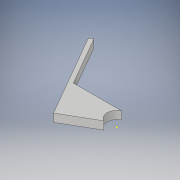
# Autodesk Inventor part: flipper-hug-left
Saved by Autodesk Inventor 2017 (Build 210142000, 142)
## iProperties
Created: 2017-02-21
Part Number: flipper-hug-left
Material: Generic
Document SubType Name: Modeling
Designer: John
Density: 1 g/cm^3
Appearance: Default
Author: John
Autodesk Inventor part; units mm, degrees
ref_plane "YZ Plane" through (0, 0, 0) normal (1, 0, 0) x (0, 1, 0)
ref_plane "XZ Plane" through (0, 0, 0) normal (0, 1, 0) x (-1, 0, 0)
ref_plane "XY Plane" through (0, 0, 0) normal (0, 0, 1) x (1, 0, 0)
sketch "Sketch1" plane through (0, 0, 0) normal (0, 1, 0) x (-1, 0, 0)
  point P0 (0, 0)
sketch "Sketch2" plane through (0, 0, 0) normal (0, 1, 0) x (-1, 0, 0)
  circle A0 centre (0, 0) radius 10 construction
  arc A1 (5.0714, -10.8757) -> (5.0714, 10.8757) centre (0, 0) ccw
  line L0 (5.0714, 10.8757) -> (5.0714, -10.8757) construction
  line L1 (5.0714, 10.8757) -> (26.8228, 10.8757) construction
  line L2 (5.0714, -10.8757) -> (65.0714, -10.8757)
  line L3 (5.0714, -10.8757) -> (65.0714, -10.8757) construction
  line L4 (65.0714, -10.8757) -> (100.0714, -71.4975)
  line L5 (100.0714, -71.4975) -> (104.4015, -68.9975)
  line L6 (5.0714, 10.8757) -> (58.2868, 10.8757)
  line L7 (58.2868, 10.8757) -> (104.4015, -68.9975)
  dimension "d0" = 20
  dimension "d1" = 90
  dimension "d2" = 2
  dimension "d3" = 130
  dimension "d4" = 60
  dimension "d5" = 0
  dimension "d6" = 70
  dimension "d7" = 120
  dimension "d8" = 5
  constraints: 16 end point, 3 horizontal, 2 centre point, 2 equal length, 2 point on circle, 1 coincident, 1 concentric, 1 parallel, 1 perpendicular, 1 point on line
  measures "d0" diameter of A0
  measures "d1" angle of L0 L1
  measures "d2" radial gap between concentric circles of A1 A0
  measures "d4" distance of L0.end L2.end
  measures "d5" distance between parallel lines of L2 L3
  measures "d6" distance of L2.end L4.end
  measures "d7" angle of L2 L4
  measures "d8" distance of L4.end L5.end
extrude "Extrusion1" add sketch "Sketch2" along normal blind 10
sketch "Sketch3" plane through (0, 10, 0) normal (0, 1, 0) x (1, 0, 0)
  line L0 (-58.2868, -10.8757) -> (-104.4015, 68.9975) projected
  line L1 (-58.2868, -10.8757) -> (-44.9829, -33.9186)
  arc A0 (-5.0714, 10.8757) -> (-5.0714, -10.8757) centre (0, 0) ccw projected
  line L2 (-44.9829, -33.9186) -> (-5.0714, -10.8757)
  line L3 (-58.2868, -10.8757) -> (-5.0714, -10.8757) projected
  line L4 (-58.2868, -10.8757) -> (-5.0714, -10.8757)
  constraints: 6 end point, 1 collinear, 1 horizontal, 1 perpendicular
extrude "Extrusion2" add sketch "Sketch3" against normal blind 10
body "Solid1"
